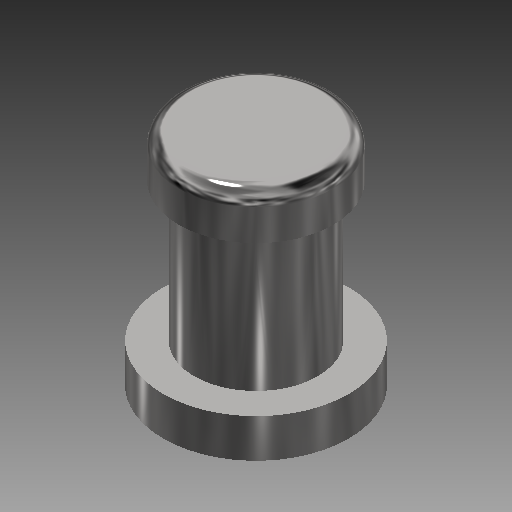
# Autodesk Inventor part: 312-02
Saved by Autodesk Inventor 2019 (Build 230136000, 136)
## iProperties
Company: Autodesk Inc.
Created: 2007-10-25
Part Number: 312-02
Document SubType Name: Modeling
Designer: Autodesk Inc.
Density: 8 g/cm^3
Mass: 7.71449 g
Surface Area: 6.83505 cm^2
Volume: 0.964311 cm^3
Material: Stainless Steel
Description: PIVOT PIN
Appearance: Steel - Polished
Component Category: Fasteners
Author: Inventor
Autodesk Inventor part; units mm, degrees
ref_plane "YZ Plane" through (0, 0, 0) normal (1, 0, 0) x (0, 1, 0)
ref_plane "XZ Plane" through (0, 0, 0) normal (0, 1, 0) x (-1, 0, 0)
ref_plane "XY Plane" through (0, 0, 0) normal (0, 0, 1) x (1, 0, 0)
sketch "Sketch1" plane through (0, 0, 0) normal (0, 0, 1) x (1, 0, 0)
  line L0 (-1.2, 0) -> (7.2, 0) projected
  line L1 (0, -9.9414) -> (0, 10.6485) projected
  line L2 (0, -7) -> (6, -7)
  line L3 (6, -7) -> (6, -4.5)
  line L4 (6, -4.5) -> (4, -4.5)
  line L5 (4, -4.5) -> (4, 4.5)
  line L6 (4, 4.5) -> (5, 4.5)
  line L7 (5, 4.5) -> (5, 6.5)
  line L8 (4, 7.5) -> (0, 7.5)
  arc A0 (5, 6.5) -> (4, 7.5) centre (4, 6.5) ccw
  point P0 (0, 0)
  point P1 (4, 0)
  dimension "d1" = 10
  dimension "d2" = 8
  dimension "d3" = 12
  dimension "d4" = 9
  dimension "d5" = 3
  dimension "d6" = 2.5
  dimension "d7" = 1
  constraints: 14 end point, 5 perpendicular, 3 point on line, 2 parallel, 2 point on circle, 2 tangent, 1 centre point, 1 midpoint
  measures "d1" diameter of L7 L1
  measures "d2" diameter of L5 L1
  measures "d3" diameter of L3 L1
  measures "d4" distance between parallel lines of L6 L4
  measures "d5" distance between parallel lines of L8 L6
  measures "d6" distance between parallel lines of L2 L4
  measures "d7" radius of A0
revolve "Revolution1" add sketch "Sketch1" angle 360 about axis through (0, -10, 0) along (0, 1, 0)
body "Solid1"
